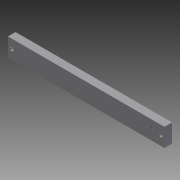
# Autodesk Inventor part: SensorBar
Saved by Autodesk Inventor 2012 (Build 160160000, 160)
## iProperties
Created: 2012-04-10
Part Number: SensorBar
Material: Default
Document SubType Name: Modeling
Designer: Admin
Density: 1 g/cm^3
Mass: 42.0977 g
Surface Area: 136.467 cm^2
Volume: 42.0977 cm^3
Author: Admin
Autodesk Inventor part; units mm, degrees
ref_plane "YZ Plane" through (0, 0, 0) normal (1, 0, 0) x (0, 1, 0)
ref_plane "XZ Plane" through (0, 0, 0) normal (0, 1, 0) x (-1, 0, 0)
ref_plane "XY Plane" through (0, 0, 0) normal (0, 0, 1) x (1, 0, 0)
sketch "Sketch1" plane through (0, 0, 0) normal (0, 0, 1) x (1, 0, 0)
  line L0 (0, 0) -> (195.58, 0)
  line L1 (195.58, 0) -> (195.58, 22.86)
  line L2 (195.58, 22.86) -> (0, 22.86)
  line L3 (0, 22.86) -> (0, 0)
  dimension "d0" = 22.86
  dimension "d1" = 195.58
  constraints: 8 end point, 2 parallel, 1 horizontal, 1 perpendicular
  measures "d0" distance of L2.end L0.start
  measures "d1" distance of L0.start L0.end
extrude "Extrusion1" add sketch "Sketch1" along normal blind 9.525
sketch "Sketch2" plane through (0, 0, 9.525) normal (0, 0, 1) x (1, 0, 0)
  line L0 (0, 34.235) -> (9.525, 34.235) projected
  line L1 (0, 0) -> (0, 34.235) projected
  line L2 (9.525, 0) -> (0, 0) projected
  line L3 (9.525, 34.235) -> (9.525, 0) projected
  line L4 (73.66, 34.235) -> (83.185, 34.235) projected
  line L5 (73.66, 0) -> (73.66, 34.235) projected
  line L6 (83.185, 0) -> (73.66, 0) projected
  line L7 (83.185, 34.235) -> (83.185, 0) projected
  line L8 (121.92, 34.235) -> (112.395, 34.235)
  line L9 (112.395, 34.235) -> (112.395, 0)
  line L10 (112.395, 0) -> (121.92, 0)
  line L11 (121.92, 0) -> (121.92, 34.235)
  line L12 (195.58, 34.235) -> (186.055, 34.235)
  line L13 (186.055, 34.235) -> (186.055, 0)
  line L14 (186.055, 0) -> (195.58, 0)
  line L15 (195.58, 0) -> (195.58, 34.235)
  circle A0 centre (77.45, 4.06) radius 1.0795 projected
  circle A1 centre (77.45, 20.36) radius 1.0795 projected
  circle A2 centre (4.7625, 11.43) radius 1.651 projected
  point P0 (4.7625, 11.43)
  point P1 (190.8175, 11.43)
  constraints: 16 end point
hole "Hole1" at (4.7625, 11.43, 9.525) at (190.8175, 11.43, 9.525) direction (0, 0, -1) diameter 4.318 end through all clearance for "Flat Head Machine Screw (82)" size "#8" standard "Ansi Unified Screw Threads"
sketch "Sketch3" plane through (0, 0, 9.525) normal (0, 0, 1) x (1, 0, 0)
  circle A0 centre (52.935, 13.82) radius 1.6 projected
  circle A1 centre (15.935, 13.82) radius 1.6 projected
  circle A2 centre (77.45, 4.06) radius 1.55 projected
  circle A3 centre (118.15, 20.36) radius 1.55 projected
  circle A4 centre (142.645, 13.82) radius 1.6 projected
  circle A5 centre (179.645, 13.82) radius 1.6 projected
  constraints: 6 coincident
hole "Hole2" at (77.45, 4.06, 9.525) at (118.15, 20.36, 9.525) at (52.935, 13.82, 9.525) at (15.935, 13.82, 9.525) at (142.645, 13.82, 9.525) at (179.645, 13.82, 9.525) direction (0, 0, -1) diameter 2.159 end through all
body "Solid1"
